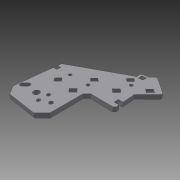
# Autodesk Inventor part: z_axis_top
Saved by Autodesk Inventor 2014 (Build 180170000, 170)
## iProperties
Created: 2013-12-06
Part Number: z_axis_top
Material: Generic
Document SubType Name: Modeling
Designer: buben
Density: 1 g/cm^3
Appearance: Anodized - Dark Gray
Author: buben
Subject: Laser Cutted
Autodesk Inventor part; units mm, degrees
ref_plane "YZ Plane" through (0, 0, 0) normal (1, 0, 0) x (0, 1, 0)
ref_plane "XZ Plane" through (0, 0, 0) normal (0, 1, 0) x (-1, 0, 0)
ref_plane "XY Plane" through (0, 0, 0) normal (0, 0, 1) x (1, 0, 0)
sketch "Sketch1" plane through (0, 0, 0) normal (0, 0, 1) x (1, 0, 0)
  line L0 (0, 0) -> (0, -52)
  line L1 (0, -52) -> (10, -62)
  line L2 (10, -62) -> (50, -62)
  line L3 (50, -62) -> (60, -52)
  line L4 (60, -52) -> (60, -6)
  line L5 (0, 0) -> (6, 0)
  line L6 (6, 0) -> (6, 6)
  line L7 (6, 6) -> (0, 6)
  line L8 (0, 6) -> (0, 12)
  line L9 (0, 12) -> (76, 50)
  line L10 (60, -6) -> (96, -6)
  line L11 (96, -6) -> (96, 0)
  line L12 (96, 0) -> (90, 0)
  line L13 (90, 0) -> (90, 6)
  line L14 (90, 6) -> (96, 6)
  line L15 (96, 6) -> (96, 50)
  line L16 (96, 50) -> (76, 50)
  circle A0 centre (49, -42) radius 2.5
  circle A1 centre (26, -42) radius 4
  dimension "d0" = 45
  dimension "d1" = 10
  dimension "d2" = 8
  dimension "d3" = 5
  dimension "d4" = 23
  dimension "d5" = 6
  dimension "d6" = 6
  dimension "d7" = 6
  dimension "d8" = 42
  dimension "d9" = 6
  dimension "d10" = 26
  dimension "d11" = 44
  dimension "d12" = 20
  dimension "d14" = 6
  dimension "d15" = 84
  dimension "d16" = 60
  dimension "d17" = 20
  constraints: 34 end point, 7 parallel, 5 collinear, 5 perpendicular, 2 centre point, 2 horizontal alignment, 1 vertical
  measures "d0" angle of L0 L1
  measures "d1" horizontal distance of L1.end L0.end
  measures "d2" diameter of A1
  measures "d3" diameter of A0
  measures "d4" distance of A1.centre A0.centre
  measures "d5" distance of L5.end L6.end
  measures "d6" distance of L0.start L5.end
  measures "d7" distance of L13.end L14.end
  measures "d8" distance from line of A1.centre L5
  measures "d9" distance of L10.end L11.end
  measures "d10" distance from line of A1.centre L0
  measures "d11" distance of L14.end L15.end
  measures "d12" distance of L15.end L9.end
  measures "d14" distance of L7.end L8.end
  measures "d15" distance between parallel lines of L13 L6
  measures "d16" distance between parallel lines of L4 L0
  measures "d17" distance from line of L2 A1.centre
extrude "Extrusion1" add sketch "Sketch1" along normal blind 6
sketch "Sketch14" plane through (0, 0, 6) normal (0, 0, 1) x (1, 0, 0)
  line L0 (0, 0) -> (0, -52) projected
  line L1 (90, 6) -> (96, 6) projected
  line L2 (96, 6) -> (96, 50) projected
  line L3 (96, 50) -> (76, 50) projected
  line L4 (6, 0) -> (0, 0) projected
  line L5 (6.5, -42) -> (116, 65) construction
  line L6 (78.114, 50) -> (93.9064, 65.4319)
  line L7 (93.9064, 65.4319) -> (115.9216, 42.9023)
  line L8 (115.9216, 42.9023) -> (96, 23.4356)
  line L9 (78.114, 50) -> (96, 50)
  line L10 (96, 50) -> (96, 23.4356)
  dimension "d101" = 6.5
  dimension "d102" = 42
  dimension "d103" = 59
  dimension "d104" = 20
  dimension "d108" = 31.5
  dimension "d109" = 15.75
  dimension "d110" = 15.5
  constraints: 12 end point, 2 collinear, 2 perpendicular, 2 point on line, 1 coincident, 1 parallel
  measures "d101" distance from line of L0 L5.start
  measures "d102" distance from line of L5.start L4
  measures "d103" distance from line of L5.end L1
  measures "d104" distance from line of L5.end L2
  measures "d108" distance between parallel lines of L8 L6
  measures "d109" distance between parallel lines of L5 L6
  measures "d110" distance from line of L7 L5.end
extrude "Extrusion11" add sketch "Sketch14" against normal blind 6
sketch "Sketch15" plane through (0, 0, 6) normal (0, 0, 1) x (1, 0, 0)
  line L0 (0, 0) -> (0, -52) projected
  line L1 (115.9216, 42.9023) -> (93.9064, 65.4319) projected
  line L2 (104.914, 54.1671) -> (0, -48.3516) construction
  line L3 (4.3543, -44.0967) -> (8.6457, -39.9033) construction
  line L4 (6.451, -46.2424) -> (10.7424, -42.049)
  line L5 (6.549, -37.7576) -> (2.2576, -41.951)
  arc A0 (2.2576, -41.951) -> (6.451, -46.2424) centre (4.3543, -44.0967) ccw
  arc A1 (10.7424, -42.049) -> (6.549, -37.7576) centre (8.6457, -39.9033) ccw
  point P0 (6.5, -42)
  point P1 (6.5, -42)
  dimension "d113" = 6.5
  dimension "d114" = 6
  dimension "d116" = 6
  constraints: 10 end point, 4 point on circle, 4 tangent, 2 centre point, 2 midpoint, 2 point on line, 1 coincident, 1 collinear, 1 parallel, 1 perpendicular
  measures "d113" distance from line of L0 point (6.5, -42)
  measures "d114" distance between parallel lines of L5 L4
  measures "d116" distance of L3.start L3.end
extrude "Extrusion12" cut sketch "Sketch15" against normal blind 6
sketch "Sketch16" plane through (0, 0, 6) normal (0, 0, 1) x (1, 0, 0)
  circle A0 centre (26, -42) radius 4 projected
  circle A1 centre (49, -42) radius 2.5 projected
  line L0 (6, 0) -> (0, 0) projected
  circle A2 centre (37.5, -36) radius 2.25
  circle A3 centre (37.5, -48) radius 2.25
  line L1 (37.5, -36) -> (37.5, -48) construction
  line L2 (26, -42) -> (49, -42) construction
  point P0 (37.5, -42)
  dimension "d119" = 4.5
  dimension "d120" = 12
  constraints: 4 end point, 2 centre point, 2 midpoint, 2 perpendicular, 1 equal radius, 1 vertical alignment
  measures "d119" diameter of A3
  measures "d120" distance of L1.start L1.end
extrude "Extrusion13" cut sketch "Sketch16" against normal through all contours A2 | A3
sketch "Sketch17" plane through (0, 0, 6) normal (0, 0, 1) x (1, 0, 0)
  line L0 (93.9064, 65.4319) -> (78.114, 50) projected
  line L1 (78.114, 50) -> (76, 50) projected
  line L2 (6, 0) -> (0, 0) projected
  line L3 (87.3242, 59) -> (78, 59)
  line L4 (78, 50) -> (78, 59)
  dimension "d124" = 2
  dimension "d125" = 9
  constraints: 4 end point, 2 point on line, 1 parallel, 1 perpendicular
  measures "d124" distance from line of L1.end L4
  measures "d125" distance of L4.start L3.end
extrude "Extrusion14" add sketch "Sketch17" against normal blind 6
sketch "Sketch18" plane through (0, 0, 6) normal (0, 0, 1) x (1, 0, 0)
  line L0 (87.3242, 59) -> (78, 59) projected
  line L1 (78, 59) -> (78, 50) projected
  line L2 (81, 56) -> (87, 56)
  line L3 (87, 56) -> (87, 50)
  line L4 (87, 50) -> (81, 50)
  line L5 (81, 50) -> (81, 56)
  dimension "d128" = 6
  dimension "d129" = 3
  dimension "d130" = 3
  constraints: 8 end point, 2 parallel, 2 perpendicular, 1 horizontal
  measures "d128" distance of L2.end L3.end
  measures "d129" distance between parallel lines of L0 L2
  measures "d130" distance between parallel lines of L1 L5
extrude "Extrusion15" cut sketch "Sketch18" against normal blind 6
sketch "Sketch19" plane through (0, 0, 6) normal (0, 0, 1) x (1, 0, 0)
  line L0 (96, 23.4356) -> (115.9216, 42.9023) projected
  line L1 (115.9216, 42.9023) -> (93.9064, 65.4319) projected
  line L2 (93.9064, 65.4319) -> (87.3242, 59) projected
  line L3 (6, 0) -> (0, 0) projected
  line L4 (78.1225, 45.8139) -> (72.4007, 40.2227)
  line L5 (72.4007, 40.2227) -> (76.5941, 35.9314)
  line L6 (76.5941, 35.9314) -> (82.3159, 41.5225)
  line L7 (82.3159, 41.5225) -> (78.1225, 45.8139)
  line L8 (50.944, 19.2559) -> (55.1374, 14.9645)
  line L9 (55.1374, 14.9645) -> (49.4156, 9.3733)
  line L10 (49.4156, 9.3733) -> (45.2222, 13.6647)
  line L11 (45.2222, 13.6647) -> (50.944, 19.2559)
  line L12 (23.7655, -7.3022) -> (27.9588, -11.5935)
  line L13 (27.9588, -11.5935) -> (22.237, -17.1847)
  line L14 (22.237, -17.1847) -> (18.0437, -12.8933)
  line L15 (18.0437, -12.8933) -> (23.7655, -7.3022)
  line L16 (6, 6) -> (90, 6) construction
  line L17 (108.1031, 39.4569) -> (103.9098, 43.7482)
  line L18 (103.9098, 43.7482) -> (98.188, 38.157)
  line L19 (98.188, 38.157) -> (102.3813, 33.8657)
  line L20 (102.3813, 33.8657) -> (108.1031, 39.4569)
  line L21 (84.5007, 16.3933) -> (80.3074, 20.6847)
  line L22 (80.3074, 20.6847) -> (74.5856, 15.0935)
  line L23 (74.5856, 15.0935) -> (78.7789, 10.8022)
  line L24 (78.7789, 10.8022) -> (84.5007, 16.3933)
  line L25 (53.7461, -13.6592) -> (49.5527, -9.3678)
  line L26 (49.5527, -9.3678) -> (43.8309, -14.959)
  line L27 (43.8309, -14.959) -> (48.0243, -19.2503)
  line L28 (48.0243, -19.2503) -> (53.7461, -13.6592)
  dimension "d133" = 8
  dimension "d134" = 6
  dimension "d135" = 3
  dimension "d136" = 25
  dimension "d137" = 30
  dimension "d138" = 30
  dimension "d139" = 3
  dimension "d140" = 8
  dimension "d141" = 25
  dimension "d142" = 35
  constraints: 50 end point, 16 parallel, 10 equal length, 9 perpendicular, 4 collinear
  measures "d133" distance of L4.start L4.end
  measures "d134" distance of L6.end L4.start
  measures "d135" distance between parallel lines of L4 L2
  measures "d136" distance between parallel lines of L1 L7
  measures "d137" distance between parallel lines of L5 L8
  measures "d138" distance between parallel lines of L12 L10
  measures "d139" distance between parallel lines of L0 L20
  measures "d140" distance between parallel lines of L1 L17
  measures "d141" distance between parallel lines of L19 L21
  measures "d142" distance between parallel lines of L25 L23
extrude "Extrusion16" cut sketch "Sketch19" against normal blind 6
sketch "Sketch20" plane through (0, 0, 6) normal (0, 0, 1) x (1, 0, 0)
  line L0 (74.5856, 15.0935) -> (80.3074, 20.6847) projected
  line L1 (82.3159, 41.5225) -> (76.5941, 35.9314) projected
  line L2 (55.1374, 14.9645) -> (49.4156, 9.3733) projected
  line L3 (87, 50) -> (81, 50) projected
  line L4 (6, 6) -> (6, 0) projected
  circle A0 centre (52.5514, 3) radius 2.25
  circle A1 centre (84, 33.7306) radius 2.25
  point P0 (6, 3)
  point P1 (84, 50)
  dimension "d145" = 4.5
  dimension "d146" = 6.75
  dimension "d147" = 13.5
  dimension "d148" = 6.75
  constraints: 2 centre point, 2 midpoint, 1 equal radius, 1 horizontal alignment, 1 vertical alignment
  measures "d145" diameter of A0
  measures "d146" distance from line of L2 A0.centre
  measures "d147" distance between parallel lines of L0 L2
  measures "d148" distance from line of L1 A1.centre
extrude "Extrusion17" cut sketch "Sketch20" against normal blind 6
sketch "Sketch21" plane through (0, 0, 6) normal (0, 0, 1) x (1, 0, 0)
  line L0 (93.9064, 65.4319) -> (87.3242, 59) projected
  line L1 (0, 12) -> (0, 6) projected
  line L2 (6, 6) -> (6, 0) projected
  circle A0 centre (25, 3) radius 2.25
  line L3 (45.2222, 13.6647) -> (23.7655, -7.3022) construction
  circle A1 centre (25, 3) radius 4.5 construction
  point P0 (6, 3)
  dimension "d151" = 25
  dimension "d152" = 4.5
  dimension "d153" = 9
  constraints: 2 centre point, 2 end point, 1 coincident, 1 horizontal alignment, 1 midpoint, 1 parallel
  measures "d151" distance from line of L1 A0.centre
  measures "d152" diameter of A0
  measures "d153" diameter of A1
extrude "Extrusion18" cut sketch "Sketch21" against normal blind 6
chamfer "Chamfer3" distance 5 angle 45 1 edges at (60, -6, 3)
chamfer "Chamfer4" distance 2 angle 45 4 edges at (96, -6, 3) (115.9216, 42.9023, 3) (93.9064, 65.4319, 3) (78, 59, 3)
body "Solid1"
